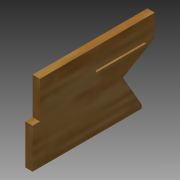
# Autodesk Inventor part: chute_wall
Saved by Autodesk Inventor 2013 (Build 170138000, 138)
## iProperties
Created: 2013-07-25
Part Number: chute_wall
Material: Generic
Document SubType Name: Modeling
Designer: dkboone
Density: 1 g/cm^3
Author: dkboone
Autodesk Inventor part; units mm, degrees
ref_plane "YZ Plane" through (0, 0, 0) normal (1, 0, 0) x (0, 1, 0)
ref_plane "XZ Plane" through (0, 0, 0) normal (0, 1, 0) x (-1, 0, 0)
ref_plane "XY Plane" through (0, 0, 0) normal (0, 0, 1) x (1, 0, 0)
sketch "Sketch1" plane through (0, 0, 0) normal (1, 0, 0) x (0, 1, 0)
  line L0 (0, 0) -> (0, -93.98)
  line L1 (0, -93.98) -> (3.175, -93.98)
  line L2 (3.175, -93.98) -> (31.2212, -77.7875)
  line L3 (31.2212, -77.7875) -> (47.0962, -105.2838)
  line L4 (47.0962, -105.2838) -> (66.04, -105.2838)
  line L5 (66.04, -105.2838) -> (66.04, -6.35)
  line L6 (34.29, 0) -> (0, 0)
  line L7 (48.26, -54.61) -> (46.6725, -54.61)
  line L8 (46.6725, -54.61) -> (46.6725, -97.79)
  line L9 (46.6725, -97.79) -> (48.26, -97.79)
  line L10 (48.26, -97.79) -> (48.26, -54.61)
  line L11 (66.04, -6.35) -> (34.29, -6.35)
  line L12 (34.29, -6.35) -> (34.29, 0)
  dimension "d2" = 31.75
  dimension "d4" = 30
  dimension "d6" = 66.04
  dimension "d7" = 93.98
  dimension "d8" = 32.385
  dimension "d9" = 3.175
  dimension "d10" = 43.18
  dimension "d11" = 1.5875
  dimension "d13" = 54.61
  dimension "d16" = 6.35
  dimension "d17" = 31.75
  dimension "d18" = 48.26
  constraints: 26 end point, 7 perpendicular, 3 parallel, 2 point on line, 1 horizontal, 1 vertical
  measures "d2" distance of L2.end L3.end
  measures "d4" angle of L0 L3
  measures "d6" distance between parallel lines of L0 L5
  measures "d7" distance of L0.start L0.end
  measures "d8" distance of L1.end L2.end
  measures "d9" distance of L0.end L1.end
  measures "d10" distance of L7.end L8.end
  measures "d11" distance of L7.start L7.end
  measures "d13" distance from line of L7.end L6
  measures "d16" distance of L11.end L6.start
  measures "d17" distance of L5.end L11.end
  measures "d18" distance between parallel lines of L0 L10
extrude "Extrusion1" add sketch "Sketch1" along normal blind 6.35
body "Solid1"
